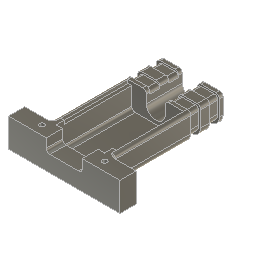
Cable PCB Mount (Autodesk Fusion 360 design; units mm, degrees)
Autodesk Fusion 360 part; units mm, degrees
sketch "Sketch1" plane through (0, 0, 0) normal (0, 0, 1) x (1, 0, 0)
  line L0 (0, 0) -> (62, 0)
  line L1 (62, 0) -> (62, 9)
  line L2 (62, 9) -> (0, 9)
  line L3 (0, 9) -> (0, 0)
  line L4 (13.5, 9) -> (48.5, 9)
  line L5 (48.5, 9) -> (48.5, 51)
  line L6 (48.5, 51) -> (13.5, 51)
  line L7 (13.5, 51) -> (13.5, 9)
  line L8 (31, 9) -> (31, 0) construction
  line L9 (31, 51) -> (31, 9) construction
  line L10 (15.5, 9) -> (15.5, 51)
  line L11 (46.5, 9) -> (46.5, 51)
  line L12 (17.5, 9) -> (17.5, 51)
  line L13 (44.5, 9) -> (44.5, 51)
  line L14 (21.75, 51) -> (40.25, 51)
  line L15 (40.25, 51) -> (40.25, 71)
  line L16 (40.25, 71) -> (21.75, 71)
  line L17 (21.75, 71) -> (21.75, 51)
  line L18 (36.25, 51) -> (36.25, 71)
  line L19 (25.75, 51) -> (25.75, 71)
  line L20 (15.5, 9) -> (46, 9)
  line L21 (46, 9) -> (46, 7)
  line L22 (46, 7) -> (15.5, 7)
  line L23 (15.5, 7) -> (15.5, 9)
  line L24 (40.25, 71) -> (48.5, 71)
  line L25 (48.5, 71) -> (48.5, 51)
  line L26 (48.5, 51) -> (40.25, 51)
  line L27 (40.25, 51) -> (40.25, 71)
  line L28 (21.75, 71) -> (13.5, 71)
  line L29 (13.5, 71) -> (13.5, 51)
  line L30 (13.5, 51) -> (21.75, 51)
  line L31 (21.75, 51) -> (21.75, 71)
  line L32 (48.5, 58.5) -> (13.5, 58.5)
  line L33 (13.5, 53) -> (48.5, 53)
  line L34 (48.5, 63.5) -> (13.5, 63.5)
  line L35 (13.5, 69) -> (48.5, 69)
  line L36 (47.5, 51) -> (47.5, 71)
  line L37 (14.5, 51) -> (14.5, 71)
  line L38 (48.5, 9) -> (48.5, 0) construction
  line L39 (13.5, 9) -> (13.5, 0) construction
  line L40 (62, 5) -> (0, 5) construction
  circle A0 centre (13.5, 5) radius 1.4
  circle A1 centre (48.5, 5) radius 1.4
  line L41 (21, 0) -> (41, 0)
  line L42 (41, 0) -> (41, 10.5)
  line L43 (41, 10.5) -> (21, 10.5)
  line L44 (21, 10.5) -> (21, 0)
  line L45 (13.5, 13.5) -> (48.5, 13.5)
  dimension "d1" = 62
  dimension "d2" = 9
  dimension "d3" = 35
  dimension "d4" = 42
  dimension "d8" = 2
  dimension "d9" = 2
  dimension "d10" = 4
  dimension "d11" = 4
  dimension "d27" = 18.5
  dimension "d28" = 20
  dimension "d29" = 9.25
  dimension "d34" = 4
  dimension "d35" = 4
  dimension "d45" = 2
  dimension "d49" = 1
  dimension "d50" = 1
  dimension "d51" = 5.5
  dimension "d52" = 2
  dimension "d53" = 5.5
  dimension "d54" = 2
  dimension "d66" = 5
  dimension "d67" = 2.8
  dimension "d68" = 2.8
  dimension "d74" = 20
  dimension "d75" = 10.5
  dimension "d76" = 10
  dimension "d80" = 4.5
  constraint horizontal L0
  constraint vertical L1
  constraint horizontal L2
  constraint vertical L3
  constraint coincident L0.start L3.end
  constraint horizontal L4
  constraint vertical L5
  constraint horizontal L6
  constraint vertical L7
  constraint coincident L2 L4.start
  constraint midpoint L4 L8.start
  constraint midpoint L0 L8.end
  constraint perpendicular L0 L8
  constraint midpoint L6 L9.start
  constraint coincident L2 L10.start
  constraint coincident L6 L10.end
  constraint perpendicular L6 L10
  constraint coincident L2 L11.start
  constraint coincident L6 L11.end
  constraint perpendicular L6 L11
  constraint coincident L2 L12.start
  constraint coincident L6 L12.end
  constraint perpendicular L6 L12
  constraint coincident L2 L13.start
  constraint coincident L6 L13.end
  constraint perpendicular L6 L13
  constraint horizontal L14
  constraint vertical L15
  constraint horizontal L16
  constraint vertical L17
  constraint coincident L6 L14.start
  constraint coincident L14 L18.start
  constraint coincident L16 L18.end
  constraint perpendicular L16 L18
  constraint coincident L6 L19.start
  constraint coincident L16 L19.end
  constraint perpendicular L16 L19
  constraint horizontal L20
  constraint vertical L21
  constraint horizontal L22
  constraint vertical L23
  constraint horizontal L24
  constraint vertical L25
  constraint horizontal L26
  constraint vertical L27
  constraint horizontal L28
  constraint vertical L29
  constraint horizontal L30
  constraint vertical L31
  constraint coincident L25 L32.start
  constraint coincident L29 L32.end
  constraint perpendicular L29 L32
  constraint coincident L29 L33.start
  constraint coincident L25 L33.end
  constraint perpendicular L25 L33
  constraint coincident L25 L34.start
  constraint coincident L29 L34.end
  constraint perpendicular L29 L34
  constraint coincident L29 L35.start
  constraint coincident L25 L35.end
  constraint perpendicular L25 L35
  constraint coincident L6 L36.start
  constraint coincident L24 L36.end
  constraint perpendicular L24 L36
  constraint coincident L30 L37.start
  constraint coincident L28 L37.end
  constraint perpendicular L28 L37
  constraint coincident L0 L38.end
  constraint perpendicular L0 L38
  constraint coincident L0 L39.end
  constraint perpendicular L0 L39
  constraint coincident L1 L40.start
  constraint coincident L3 L40.end
  constraint perpendicular L3 L40
  constraint coincident L39 A0.centre
  constraint coincident L40 A0.centre
  constraint coincident L40 A1.centre
  constraint coincident L38 A1.centre
  constraint horizontal L41
  constraint vertical L42
  constraint horizontal L43
  constraint vertical L44
  constraint coincident L0 L41.start
  constraint coincident L7 L45.start
  constraint coincident L5 L45.end
  constraint perpendicular L5 L45
  measures "d1" distance of L0.start L0.end
  measures "d2" distance of L0.start L2.end
  measures "d3" distance of L4.start L4.end
  measures "d4" distance of L4.start L6.end
  measures "d8" distance of L5 L11
  measures "d9" distance of L7 L10
  measures "d10" distance of L5 L13
  measures "d11" distance of L7 L12
  measures "d27" distance of L14.start L14.end
  measures "d28" distance of L14.start L16.end
  measures "d29" distance of L9 L17
  measures "d34" distance of L17 L19
  measures "d35" distance of L15 L18
  measures "d45" distance of L10.start L22.end
  measures "d49" distance of L29 L37
  measures "d50" distance of L25 L36
  measures "d51" distance of L34 L35
  measures "d52" distance of L16 L35
  measures "d53" distance of L32 L33
  measures "d54" distance of L6 L33
  measures "d66" distance of L0 L40
  measures "d67" diameter of A0
  measures "d68" diameter of A1
  measures "d74" distance of L41.start L41.end
  measures "d75" distance of L41.start L43.end
  measures "d76" distance of L8 L42
  measures "d80" distance of L20 L45
extrude "Extrude1" add sketch "Sketch1" along normal blind 16 contours L0 L2 L3 L4 L22 L23 L44 | L0 L22 L41 L42 L44 | L0 L1 L2 L4 L21 L22 L42 | L2 L4 L20 L22 L42 L44 | L2 L4 L20 L22 L23 L44 | L2 L4 L20 L21 L22 L42 | A0 | A1
extrude "Extrude2" add sketch "Sketch1" along normal blind 2 contours L2 L4 L7 L10 L45 | L2 L4 L20 L42 L43 L44 | L2 L4 L12 L13 L20 L42 L43 L44 L45 | L2 L4 L10 L12 L20 L45 | L6 L7 L10 L30 L45 | L6 L10 L12 L30 L45 | L2 L4 L5 L11 L45 | L2 L4 L11 L13 L20 L45 | L6 L12 L13 L14 L26 L30 L45 | L5 L6 L11 L26 L45 | L6 L11 L13 L26 L45
extrude "Extrude5" add sketch "Sketch1" along normal up to surface (16 mm away) contours L2 L4 L7 L10 L45 | L2 L4 L10 L12 L20 L45 | L6 L7 L10 L30 L45 | L6 L10 L12 L30 L45 | L2 L4 L5 L11 L45 | L2 L4 L11 L13 L20 L45 | L5 L6 L11 L26 L45 | L6 L11 L13 L26 L45
extrude "Extrude6" cut sketch "Sketch1" along normal blind 2 from surface at 14 contours L6 L10 L12 L30 L45 | L6 L11 L13 L26 L45
extrude "Extrude7" add sketch "Sketch1" along normal blind 4 contours L6 L14 L17 L19 L31 L33 | L17 L19 L31 L32 L33 | L6 L14 L15 L18 L27 L33 | L6 L14 L18 L19 L33 | L17 L19 L31 L32 L34 | L18 L19 L32 L33 | L15 L18 L27 L32 L33 | L17 L19 L31 L34 L35 | L18 L19 L32 L34 | L15 L18 L27 L32 L34 | L16 L17 L19 L31 L35 | L18 L19 L34 L35 | L15 L18 L27 L34 L35 | L16 L18 L19 L35 | L15 L16 L18 L27 L35
extrude "Extrude8" add sketch "Sketch1" along normal blind 16 contours L6 L29 L30 L33 L37 | L6 L17 L30 L31 L33 L37 | L29 L32 L33 L37 | L17 L31 L32 L33 L37 | L29 L32 L34 L37 | L6 L25 L26 L33 L36 | L6 L15 L26 L27 L33 L36 | L6 L14 L17 L19 L31 L33 | L17 L19 L31 L32 L33 | L17 L31 L32 L34 L37 | L29 L34 L35 L37 | L25 L32 L33 L36 | L6 L14 L15 L18 L27 L33 | L17 L19 L31 L32 L34 | L17 L31 L34 L35 L37 | L28 L29 L35 L37 | L15 L27 L32 L33 L36 | L25 L32 L34 L36 | L15 L18 L27 L32 L33 | L17 L19 L31 L34 L35 | L17 L28 L31 L35 L37 | L15 L27 L32 L34 L36 | L25 L34 L35 L36 | L15 L18 L27 L32 L34 | L16 L17 L19 L31 L35 | L15 L27 L34 L35 L36 | L24 L25 L35 L36 | L15 L18 L27 L34 L35 | L15 L24 L27 L35 L36 | L15 L16 L18 L27 L35
extrude "Extrude10" cut sketch "Sketch1" along normal up to surface (16 mm away) contours L29 L32 L33 L37 | L29 L34 L35 L37 | L25 L32 L33 L36 | L25 L34 L35 L36
extrude "Extrude11" cut sketch "Sketch1" against normal blind 1 from surface at 16 contours L17 L31 L32 L33 L37 | L17 L19 L31 L32 L33 | L18 L19 L32 L33 | L17 L31 L34 L35 L37 | L15 L27 L32 L33 L36 | L15 L18 L27 L32 L33 | L17 L19 L31 L34 L35 | L18 L19 L34 L35 | L15 L27 L34 L35 L36 | L15 L18 L27 L34 L35
extrude "Extrude12" cut sketch "Sketch1" along normal blind 1 contours L17 L31 L32 L33 L37 | L17 L19 L31 L32 L33 | L18 L19 L32 L33 | L17 L31 L34 L35 L37 | L15 L27 L32 L33 L36 | L15 L18 L27 L32 L33 | L17 L19 L31 L34 L35 | L18 L19 L34 L35 | L15 L27 L34 L35 L36 | L15 L18 L27 L34 L35
extrude "Extrude13" cut sketch "Sketch1" along normal up to surface (16 mm away) contours A0 | A1
extrude "Extrude14" cut sketch "Sketch1" against normal blind 7 from surface at 16 contours L0 L22 L41 L42 L44 | L2 L4 L20 L22 L42 L44
fillet "Fillet3" radius 5.25 2 edges at (36.25, 61, 4) (25.75, 61, 4)
fillet "Fillet4" radius 2 2 edges at (44.5, 30, 2) (17.5, 30, 2)
fillet "Fillet4" radius 2 2 edges at (21, 4.5, 9) (41, 4.5, 9)
fillet "Fillet6" radius 5.25 10 edges at (48.5, 31, 0) (47.5, 55.75, 1) (48.5, 61, 0) (47.5, 66.25, 1) (48.5, 70, 0) (13.5, 70, 0) (14.5, 66.25, 1) (13.5, 61, 0) (14.5, 55.75, 1) (13.5, 31, 0)
fillet "Fillet7" radius 2 10 edges at (48.5, 31, 16) (47.5, 55.75, 15) (48.5, 61, 16) (47.5, 66.25, 15) (48.5, 70, 16) (13.5, 70, 16) (14.5, 66.25, 15) (13.5, 61, 16) (14.5, 55.75, 15) (13.5, 31, 16)
fillet "Fillet7" radius 2 10 edges at (25.75, 52, 16) (25.75, 55.75, 15) (25.75, 61, 16) (25.75, 66.25, 15) (25.75, 70, 16) (36.25, 70, 16) (36.25, 66.25, 15) (36.25, 61, 16) (36.25, 55.75, 15) (36.25, 52, 16)
fillet "Fillet8" radius 2 6 edges at (46.9623, 9, 1.5377) (48.5, 9, 9.625) (47.9142, 9, 15.4142) (14.0858, 9, 15.4142) (13.5, 9, 9.625) (15.0377, 9, 1.5377)
